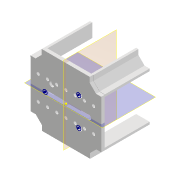
# Autodesk Inventor part: 20_Cube_insert_AlliedVision_Alvium_v3
Saved by Autodesk Inventor 2022 (Build 260153000, 153)
## iProperties
Created: 2019-08-07
Part Number: 20_Cube_insert_AlliedVision_Alvium_v3
Material: Generic
Document SubType Name: Modeling
Designer: marsikovabarbora
Density: 1 g/cm^3
Appearance: Default
Sheet Metal Rule: Standard
Author: marsikovabarbora
Autodesk Inventor part; units mm, degrees
ref_plane "Work Plane1" through (-29.1, -14.5, 2.4) normal (0, 0, -1) x (0, 1, 0)
ref_plane "Work Plane2" through (-13.8999, -10.5497, 2.25) normal (0, 0, -1) x (0, 1, 0)
ref_plane "Work Plane4" through (-17.3325, -17.0101, 2.3331) normal (0.0023441, 0.0023441, -0.9999945) x (-0.0000027, 0.9999973, 0.0023441)
sketch "Sketch1" plane through (0, 0, 0) normal (0, 0, 1) x (1, 0, 0)
  line L0 (-34.86, 0) -> (34.86, 0) construction
  line L1 (0, -34.86) -> (0, 34.86) construction
  line L2 (0, 0) -> (11.1575, 11.1575) construction
  line L3 (0, 0) -> (15.7791, 0) construction
  line L4 (0, 24.9) -> (16.8009, 24.9)
  line L5 (16.8009, 24.9) -> (16.8009, 21.2415)
  line L6 (16.8009, 21.2415) -> (19.0212, 19.0212)
  line L7 (24.9, 0) -> (24.9, 16.8009)
  line L8 (24.9, 16.8009) -> (21.2415, 16.8009)
  line L9 (21.2415, 16.8009) -> (19.0212, 19.0212)
  line L10 (0, -24.9) -> (16.8009, -24.9)
  line L11 (16.8009, -24.9) -> (16.8009, -21.2415)
  line L12 (16.8009, -21.2415) -> (19.0212, -19.0212)
  line L13 (24.9, 0) -> (24.9, -16.8009)
  line L14 (24.9, -16.8009) -> (21.2415, -16.8009)
  line L15 (21.2415, -16.8009) -> (19.0212, -19.0212)
  line L16 (0, 24.9) -> (-16.8009, 24.9)
  line L17 (-16.8009, 24.9) -> (-16.8009, 21.2415)
  line L18 (-16.8009, 21.2415) -> (-19.0212, 19.0212)
  line L19 (-24.9, 16.8009) -> (-21.2415, 16.8009)
  line L20 (-21.2415, 16.8009) -> (-19.0212, 19.0212)
  line L21 (0, -24.9) -> (-16.8009, -24.9)
  line L22 (-16.8009, -24.9) -> (-16.8009, -21.2415)
  line L23 (-16.8009, -21.2415) -> (-19.0212, -19.0212)
  line L24 (-21.2415, -16.8009) -> (-19.0212, -19.0212)
  line L25 (-24.9, -16.8009) -> (-21.2415, -16.8009)
  line L26 (-24.9, 0) -> (-24.9, -16.8009)
  line L27 (-24.9, 0) -> (-24.9, 16.8009)
  circle A0 centre (0, 0) radius 10
  dimension "d0" = 45
  dimension "d2" = 24.9
  dimension "d3" = 3.14
  dimension "d4" = 26.9
  dimension "d5" = 20
  constraints: 52 end point, 20 symmetric about line, 2 horizontal, 2 perpendicular, 2 point on line, 1 centre point, 1 coincident, 1 equal length
  measures "d0" angle of L3 L2
  measures "d2" distance between parallel lines of L0 L4
  measures "d3" distance of L5.end L6.end
  measures "d4" distance from line of L2.start L6
  measures "d5" diameter of A0
extrude "Extrusion1" add sketch "Sketch1" along normal blind 1 contours L4 L5 L6 L9 L8 L7 L13 L14 L15 L12 L11 L10 L21 L22 L23 L24 L25 L26 L27 L19 L20 L18 L17 L16 | A0
sketch "Sketch5" plane through (0, 0, 0) normal (0, 0, -1) x (-1, 0, 0)
  circle A0 centre (-9.7, 10) radius 1.4
  circle A1 centre (-9.7, -10) radius 1.4
  circle A2 centre (13.8, 0) radius 1.4
  circle A3 centre (-10, 6.9) radius 0.75
  circle A4 centre (10, 6.9) radius 1.25
  point P0 (0, 0)
  constraints: 5 centre point, 10 other
hole "Hole1" at (-13.8, 0, 0) at (9.7, -10, 0) at (9.7, 10, 0) direction (0, 0, 1) diameter 3.3 depth 12 tip angle 118
sketch "Skizze6" plane through (-16.8009, 24.9, 1) normal (0, 0, 1) x (1, 0, 0)
  circle A0 centre (6.8009, -18) radius 1.65 construction
  circle A1 centre (3.0009, -24.9) radius 1.65 construction
  circle A2 centre (26.5009, -34.9) radius 1.65 construction
  circle A3 centre (26.5009, -14.9) radius 1.65 construction
  line L0 (33.6017, -3.6585) -> (33.6017, 0) projected
  line L1 (33.6017, 0) -> (0, 0) construction
  line L2 (0, 0) -> (0, -3.6585) projected
  line L3 (0, -3.6585) -> (-4.4406, -8.0991) projected
  line L4 (-4.4406, -8.0991) -> (-8.0991, -8.0991) projected
  line L5 (-8.0991, -8.0991) -> (-8.0991, -41.7009) construction
  line L6 (-8.0991, -41.7009) -> (-4.4406, -41.7009) projected
  line L7 (-4.4406, -41.7009) -> (0, -46.1415) projected
  line L8 (0, -46.1415) -> (0, -49.8) projected
  line L9 (0, -49.8) -> (33.6017, -49.8) construction
  line L10 (33.6017, -49.8) -> (33.6017, -46.1415) projected
  line L11 (33.6017, -46.1415) -> (38.0423, -41.7009) projected
  line L12 (38.0423, -41.7009) -> (41.7009, -41.7009) projected
  line L13 (41.7009, -41.7009) -> (41.7009, -8.0991) construction
  line L14 (41.7009, -8.0991) -> (38.0423, -8.0991) projected
  line L15 (38.0423, -8.0991) -> (33.6017, -3.6585) projected
  line L16 (-0.2, 0.2) -> (33.8017, 0.2) construction
  line L17 (33.8017, 0.2) -> (33.8017, -3.5757)
  line L18 (33.8017, -3.5757) -> (38.1252, -7.8991)
  line L19 (38.1252, -7.8991) -> (41.9009, -7.8991)
  line L20 (41.9009, -7.8991) -> (41.9009, -41.9009) construction
  line L21 (41.9009, -41.9009) -> (38.1252, -41.9009)
  line L22 (38.1252, -41.9009) -> (33.8017, -46.2243)
  line L23 (33.8017, -46.2243) -> (33.8017, -50)
  line L24 (33.8017, -50) -> (-0.2, -50) construction
  line L25 (-0.2, -50) -> (-0.2, -46.2243)
  line L26 (-0.2, -46.2243) -> (-4.5235, -41.9009)
  line L27 (-4.5235, -41.9009) -> (-8.2991, -41.9009)
  line L28 (-8.2991, -41.9009) -> (-8.2991, -7.8991) construction
  line L29 (-8.2991, -7.8991) -> (-4.5235, -7.8991)
  line L30 (-4.5235, -7.8991) -> (-0.2, -3.5757)
  line L31 (-0.2, -3.5757) -> (-0.2, 0.2)
  line L32 (-8.0991, -8.0991) -> (-8.0991, -7.8991)
  line L33 (0, 0) -> (-0.2, 0)
  line L34 (33.6017, 0) -> (33.8017, 0)
  line L35 (41.7009, -8.0991) -> (38.0423, -8.0991) projected
  line L36 (41.7009, -8.0991) -> (41.7009, -7.8991)
  line L37 (41.7009, -41.7009) -> (41.7009, -41.9009)
  line L38 (33.6017, -49.8) -> (33.8017, -49.8)
  line L39 (-8.0991, -41.7009) -> (-8.0991, -41.9009)
  line L40 (0, -49.8) -> (-0.2, -49.8)
  point P0 (16.8009, -24.9)
  dimension "d25" = 0.2
  constraints: 48 end point, 12 point on line, 4 perpendicular, 15 other
  measures "d25" distance between parallel lines of L1 L16
extrude "IM_offset" add sketch "Skizze6" against normal blind 1 contours L2 L3 L4 L32 L29 L30 L31 L33 | L6 L7 L8 L40 L25 L26 L27 L39 | L10 L11 L12 L37 L21 L22 L23 L38
sketch "Sketch7" plane through (-24.9, 16.9009, 1) normal (0, 0, 1) x (1, 0, 0)
  circle A0 centre (11.1, -16.9009) radius 1.65
  line L0 (11.1, -16.9009) -> (40.9762, -16.9009) construction
  line L1 (11.1, -18.3509) -> (40.9762, -18.3509)
  line L2 (40.9762, -15.4509) -> (11.1, -15.4509)
  arc A1 (11.1, -15.4509) -> (11.1, -18.3509) centre (11.1, -16.9009) ccw
  arc A2 (40.9762, -18.3509) -> (40.9762, -15.4509) centre (40.9762, -16.9009) ccw
  circle A3 centre (40.9762, -16.9009) radius 1.65
  point P0 (24.9, -16.9009)
  point P1 (26.0381, -16.9009)
  dimension "d28" = 2.9
  constraints: 8 end point, 4 centre point, 4 point on circle, 4 tangent, 1 horizontal, 1 midpoint, 1 parallel
  measures "d28" diameter of A2
extrude "Extrusion6" cut sketch "Sketch7" against normal blind 10 contours A0 L1 A1 L2 | A0 L2 A3 L1 | A3 L1 A2 L2 | L2 A2 L1 A3 picked at (11.65, -16.9009)
ref_plane "Work Plane3" through (-24.85, -16.97, -31.85) normal (0, 0, 1) x (1, 0, 0)
sketch "Sketch9" plane through (0, 0, 0) normal (0, 0, -1) x (-1, 0, 0)
  line L0 (21.2815, 17.0009) -> (17.0009, 21.2829)
  line L1 (17.0009, 21.2829) -> (17.0009, 24.9)
  line L2 (24.9, 17.0009) -> (21.2815, 17.0009)
  line L3 (17.0009, 24.9) -> (-16.8009, 24.9) projected
  line L4 (24.9, 15.4009) -> (15.4009, 15.4009)
  line L5 (15.4009, 15.4009) -> (15.4009, 24.9)
  line L6 (15.4009, 24.9) -> (17.0009, 24.9)
  line L7 (24.9, 17.0009) -> (24.9, 15.4009)
  line L8 (24.9, 17.0009) -> (21.3243, 17.0009) projected
  line L9 (24.9, -17.0009) -> (24.9, 17.0009) projected
  line L10 (24.5679, -5) -> (24.5679, 5) construction
  line L11 (24.7337, -22.85) -> (24.7337, 22.85) construction
  line L12 (-25.1669, -24.85) -> (16.933, -24.85) construction
  line L13 (24.7325, 24.85) -> (-24.9674, 24.85) construction
  line L14 (-17.0009, -24.9) -> (17.0009, -24.9) construction
  circle A0 centre (0, 0) radius 24.9 construction
  line L15 (-24.9, 15.4009) -> (-24.9, 17.0009)
  line L16 (-21.2829, 17.0009) -> (-24.9, 17.0009)
  line L17 (-15.4009, 15.4009) -> (-24.9, 15.4009)
  line L18 (-17.0009, 21.2815) -> (-21.2829, 17.0009)
  line L19 (-17.0009, 24.9) -> (-17.0009, 21.2815)
  line L20 (-17.0009, 24.9) -> (-15.4009, 24.9)
  line L21 (-15.4009, 24.9) -> (-15.4009, 15.4009)
  line L22 (-15.4009, -24.9) -> (-17.0009, -24.9)
  line L23 (-17.0009, -21.2829) -> (-17.0009, -24.9)
  line L24 (-15.4009, -15.4009) -> (-15.4009, -24.9)
  line L25 (-21.2815, -17.0009) -> (-17.0009, -21.2829)
  line L26 (-24.9, -17.0009) -> (-21.2815, -17.0009)
  line L27 (-24.9, -17.0009) -> (-24.9, -15.4009)
  line L28 (-24.9, -15.4009) -> (-15.4009, -15.4009)
  line L29 (24.9, -15.4009) -> (24.9, -17.0009)
  line L30 (21.2829, -17.0009) -> (24.9, -17.0009)
  line L31 (15.4009, -15.4009) -> (24.9, -15.4009)
  line L32 (17.0009, -21.2815) -> (21.2829, -17.0009)
  line L33 (17.0009, -24.9) -> (17.0009, -21.2815)
  line L34 (17.0009, -24.9) -> (15.4009, -24.9)
  line L35 (15.4009, -24.9) -> (15.4009, -15.4009)
  point P0 (0, 0)
  point P1 (-24.85, 24.7325)
  point P2 (-22.85, 24.7337)
  point P3 (-17.0009, 21.3243)
  point P4 (-24.7325, -24.85)
  point P5 (-24.7337, -22.85)
  point P6 (-21.3243, -17.0009)
  point P7 (24.85, -24.7325)
  point P8 (22.85, -24.7337)
  point P9 (17.0009, -21.3243)
  point P10 (24.9, -15.4009)
  point P11 (-15.4009, 24.9)
  point P12 (-16.8009, 24.9)
  dimension "d44" = 1.6
  dimension "d64" = 1.6
  dimension "d67" = 360
  constraints: 60 end point, 5 point on line, 3 parallel, 3 tangent, 2 vertical, 1 centre point, 1 collinear, 1 horizontal, 1 perpendicular, 77 other
  measures "d44" distance of L5.end L6.end
  measures "d64" distance between parallel lines of L8 L4
ref_plane "Work Plane5" through (-25.1325, -16.9302, -31.7852) normal (-0.0023441, -0.0023441, 0.9999945) x (0.9999973, -0.0000027, 0.0023441)
extrude "Extrusion9" add sketch "Sketch9" along normal blind 31.5
ref_plane "Work Plane6" through (-16.5464, -17.0101, 2.3349) normal (0.0023441, 0.0023441, -0.9999945) x (-0.0000027, 0.9999973, 0.0023441)
sketch "Sketch11" plane through (0, 0, 1) normal (0, 0, 1) x (1, 0, 0)
  circle A0 centre (-10, 6.9) radius 1.65 projected
  circle A1 centre (9.7, 10) radius 1.65 projected
  circle A2 centre (9.7, -10) radius 1.65 projected
  arc A3 (-13.0126, 1.45) -> (-13.0126, -1.45) centre (-13.8, 0) ccw projected
  line L0 (-13.0126, 1.45) -> (15.2888, 1.45) projected
  line L1 (15.2888, -1.45) -> (-13.0126, -1.45) projected
  arc A4 (15.2888, -1.45) -> (15.2888, 1.45) centre (16.0762, 0) ccw projected
  line L2 (16.8009, 24.9) -> (-17.0009, 24.9) projected
  line L3 (-17.0009, 24.9) -> (-17.0009, 21.3243) projected
  line L4 (-17.0009, 21.3243) -> (-21.3243, 17.0009) projected
  line L5 (-21.3243, 17.0009) -> (-24.9, 17.0009) projected
  line L6 (-24.9, 17.0009) -> (-24.9, -17.0009) projected
  line L7 (-24.9, -17.0009) -> (-21.3243, -17.0009) projected
  line L8 (-21.3243, -17.0009) -> (-17.0009, -21.3243) projected
  line L9 (-17.0009, -21.3243) -> (-17.0009, -24.9) projected
  line L10 (-17.0009, -24.9) -> (17.0009, -24.9) projected
  line L11 (17.0009, -24.9) -> (17.0009, -21.3243) projected
  line L12 (17.0009, -21.3243) -> (21.3243, -17.0009) projected
  line L13 (21.3243, -17.0009) -> (24.9, -17.0009) projected
  line L14 (24.9, -17.0009) -> (24.9, 16.8009) projected
  line L15 (24.9, 16.8009) -> (21.2415, 16.8009) projected
  line L16 (21.2415, 16.8009) -> (16.8009, 21.2415) projected
  line L17 (16.8009, 21.2415) -> (16.8009, 24.9) projected
  circle A5 centre (9.7, 10) radius 1.65 projected
  circle A6 centre (9.7, -10) radius 1.65 projected
  line L18 (-13.0126, 1.45) -> (15.2888, 1.45) projected
  arc A7 (15.2888, -1.45) -> (15.2888, 1.45) centre (16.0762, 0) ccw projected
  line L19 (15.2888, -1.45) -> (-13.0126, -1.45) projected
  arc A8 (-13.0126, 1.45) -> (-13.0126, -1.45) centre (-13.8, 0) ccw projected
  point P0 (0, 0)
ref_plane "Work Plane7" through (-24.4263, -24.8901, 2.298) normal (0.0023441, 0.0023441, -0.9999945) x (-0.0000027, 0.9999973, 0.0023441)
extrude "Extrusion11" add sketch "Sketch11" along normal up to surface surface through (-24.4263, -24.8901, 2.298) normal (0.0023441, 0.0023441, -0.9999945)
sketch "Sketch12" plane through (-24.9, -17.0009, 2.3154) normal (-0.0023441, -0.0023441, 0.9999945) x (0.9999973, -0.0000055, 0.0023441)
  ellipse E0 centre (33.8151, 6.927) end of major axis (35.3151, 6.927) minor radius 1.5
  ellipse E1 centre (33.8151, 26.9269) end of major axis (35.3151, 26.9269) minor radius 1.5
  ellipse E2 centre (10.1152, 16.9269) end of major axis (11.6152, 16.9269) minor radius 1.5
  point P0 (24.8944, 16.9954)
  constraints: 3 centre point, 6 other
ref_plane "Arbeitsebene8" through (-14.96, 0, 0) normal (0, -1, 0) x (1, 0, 0)
ref_plane "Arbeitsebene9" through (0, -14.96, 0) normal (1, 0, 0) x (0, 0, -1)
sketch "Skizze13" plane through (0, 0, 0) normal (0, 0, -1) x (-1, 0, 0)
  line L0 (-15.4009, -24.9) -> (15.4009, -24.9) projected
  line L1 (24.9, -15.4009) -> (24.9, 15.4009) projected
  line L2 (15.4009, 24.9) -> (-15.4009, 24.9) projected
  line L3 (-24.9, 15.4009) -> (-24.9, -15.4009) projected
  line L4 (-15.2888, 1.45) -> (13.0126, 1.45) projected
  arc A0 (13.0126, -1.45) -> (13.0126, 1.45) centre (13.8, 0) ccw projected
  line L5 (13.0126, -1.45) -> (-15.2888, -1.45) projected
  arc A1 (-15.2888, 1.45) -> (-15.2888, -1.45) centre (-16.0762, 0) ccw projected
  circle A2 centre (-9.7, -10) radius 1.65 projected
  circle A3 centre (-9.7, 10) radius 1.65 projected
  circle A4 centre (0.0204, 8.5) radius 1.1
  circle A5 centre (0.0204, -8.5) radius 1.1
  line L6 (-21.3243, -17.0009) -> (-17.0009, -21.3243) projected
  line L7 (17.0009, -21.3243) -> (21.3243, -17.0009) projected
  line L8 (21.3243, 17.0009) -> (17.0009, 21.3243) projected
  line L9 (-15.4009, -15.4009) -> (-15.4009, -24.9) projected
  line L10 (15.4009, -24.9) -> (15.4009, -15.4009) projected
  line L11 (15.4009, -15.4009) -> (24.9, -15.4009) projected
  line L12 (24.9, 15.4009) -> (15.4009, 15.4009) projected
  line L13 (15.4009, 15.4009) -> (15.4009, 24.9) projected
  line L14 (-15.4009, 24.9) -> (-15.4009, 15.4009) projected
  line L15 (-15.4009, 15.4009) -> (-24.9, 15.4009) projected
  line L16 (-24.9, -15.4009) -> (-15.4009, -15.4009) projected
  line L17 (-17.0009, -21.3243) -> (-17.0009, -21.2829) projected
  line L18 (-17.0009, -21.2829) -> (-21.2815, -17.0009) projected
  line L19 (-21.2815, -17.0009) -> (-21.3243, -17.0009) projected
  line L20 (17.0009, -21.2815) -> (17.0009, -21.3243) projected
  line L21 (21.3243, -17.0009) -> (21.2829, -17.0009) projected
  line L22 (21.2829, -17.0009) -> (17.0009, -21.2815) projected
  line L23 (17.0009, 21.3243) -> (17.0009, 21.2829) projected
  line L24 (17.0009, 21.2829) -> (21.2815, 17.0009) projected
  line L25 (21.2815, 17.0009) -> (21.3243, 17.0009) projected
  point P0 (0, 0)
  dimension "d55" = 2.2
  dimension "d56" = 2.2
  dimension "d57" = 8.5
  dimension "d58" = 8.5
  constraints: 2 centre point
  measures "d55" diameter of A4
  measures "d56" diameter of A5
  measures "d57" vertical distance of A4.centre point (0, 0)
  measures "d58" vertical distance of point (0, 0) A5.centre
extrude "Extrusion12" cut sketch "Skizze13" against normal blind 31.5 contours A4 | A5
pattern_linear "Rechteckige Anordnung1" count 7 spacing 6.5 along (1, 0, 0) of "Extrusion12" first direction both ways yes
equation "\"d44\" = d64"
equation "\"BendRadius\" = Thickness"
equation "\"BendReliefWidth\" = Thickness"
equation "\"BendReliefDepth\" = 0.5 * Thickness"
equation "\"CornerReliefSize\" = 4 * Thickness"
equation "\"MinimumRemnant\" = 2 * Thickness"
equation "\"TransitionRadius\" = BendRadius"
equation "\"JacobiRadiusSize\" = Thickness"
equation "\"GapSize\" = Thickness"
equation "\"Thickness\" = 0.5"
body "Solid1"
